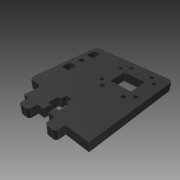
# Autodesk Inventor part: x_motor_cable_mount
Saved by Autodesk Inventor 2014 (Build 180170000, 170)
## iProperties
Created: 2013-12-02
Part Number: x_motor_cable_mount
Material: Plywood, Finish
Document SubType Name: Modeling
Designer: buben
Density: 0.552 g/cm^3
Appearance: Plywood - New
Author: buben
Subject: Laser Cutted
Autodesk Inventor part; units mm, degrees
ref_plane "YZ Plane" through (0, 0, 0) normal (1, 0, 0) x (0, 1, 0)
ref_plane "XZ Plane" through (0, 0, 0) normal (0, 1, 0) x (-1, 0, 0)
ref_plane "XY Plane" through (0, 0, 0) normal (0, 0, 1) x (1, 0, 0)
sketch "Sketch1" plane through (0, 0, 0) normal (0, 0, 1) x (1, 0, 0)
  line L0 (12.2, 0) -> (64.2, 0)
  line L1 (64.2, 0) -> (64.2, 72)
  line L2 (64.2, 72) -> (0, 72)
  line L3 (0, 72) -> (0, 12)
  line L4 (3, 66) -> (9.5, 66)
  line L5 (9.5, 66) -> (9.5, 58)
  line L6 (9.5, 58) -> (3, 58)
  line L7 (3, 58) -> (3, 66)
  line L8 (3, 43) -> (9.5, 43)
  line L9 (9.5, 43) -> (9.5, 35)
  line L10 (9.5, 35) -> (3, 35)
  line L11 (3, 35) -> (3, 43)
  line L12 (0, 12) -> (12.2, 12)
  line L13 (12.2, 12) -> (12.2, 0)
  line L14 (3, 58) -> (9.5, 43) construction
  line L15 (3, 43) -> (9.5, 58) construction
  circle A0 centre (6.25, 50.5) radius 2.25
  point P0 (0, 0)
  dimension "d1" = 6.5
  dimension "d2" = 8
  dimension "d3" = 8
  dimension "d4" = 15
  dimension "d5" = 3
  dimension "d6" = 72
  dimension "d7" = 4.5
  dimension "d8" = 64.2
  dimension "d9" = 12
  dimension "d10" = 52
  dimension "d11" = 6
  constraints: 32 end point, 6 parallel, 5 perpendicular, 3 horizontal, 2 collinear, 1 centre point, 1 horizontal alignment, 1 midpoint, 1 vertical alignment
  measures "d1" distance of L4.start L4.end
  measures "d2" distance of L4.end L5.end
  measures "d3" distance of L8.end L9.end
  measures "d4" distance between parallel lines of L6 L8
  measures "d5" distance between parallel lines of L3 L7
  measures "d6" distance between parallel lines of L0 L2
  measures "d7" diameter of A0
  measures "d8" distance between parallel lines of L1 L3
  measures "d9" distance of L12.end L0.start
  measures "d10" distance of L0.start L0.end
  measures "d11" distance between parallel lines of L2 L4
extrude "Extrusion1" add sketch "Sketch1" along normal blind 6.5
sketch "Sketch2" plane through (0, 0, 6.5) normal (0, 0, 1) x (1, 0, 0)
  line L0 (64.2, 0) -> (64.2, 72) projected
  line L1 (12.2, 0) -> (64.2, 0) projected
  line L2 (29.95, 16.3) -> (34.45, 16.3)
  line L3 (34.45, 0) -> (29.95, 0)
  line L4 (36.95, 12.3) -> (36.95, 5)
  line L5 (27.45, 5) -> (27.45, 12.3)
  line L6 (29.95, 0) -> (29.95, 5)
  line L7 (29.95, 12.3) -> (29.95, 16.3)
  line L8 (27.45, 12.3) -> (29.95, 12.3)
  line L9 (34.45, 12.3) -> (36.95, 12.3)
  line L10 (34.45, 16.3) -> (34.45, 12.3)
  line L11 (34.45, 5) -> (34.45, 0)
  line L12 (36.95, 5) -> (34.45, 5)
  line L13 (29.95, 5) -> (27.45, 5)
  point P0 (0, 0)
  point P1 (32.2, 16.3)
  dimension "d14" = 2.5
  dimension "d15" = 2.5
  dimension "d16" = 4.5
  dimension "d17" = 5
  dimension "d18" = 7.3
  dimension "d19" = 4
  dimension "d20" = 32
  constraints: 24 end point, 10 parallel, 5 collinear, 4 perpendicular, 3 horizontal, 1 midpoint
  measures "d14" distance of L5.end L7.start
  measures "d15" distance of L9.start L4.start
  measures "d16" distance of L2.start L2.end
  measures "d17" distance of L11.start L3.start
  measures "d18" distance of L4.start L4.end
  measures "d19" distance of L2.end L9.start
  measures "d20" distance from line of L0 point (32.2, 16.3)
extrude "Extrusion2" cut sketch "Sketch2" against normal blind 6.5
sketch "Sketch3" plane through (0, 0, 6.5) normal (0, 0, 1) x (1, 0, 0)
  line L0 (34.45, 0) -> (64.2, 0) projected
  line L1 (12.2, 0) -> (29.95, 0) projected
  line L2 (29.95, 16.3) -> (34.45, 16.3) projected
  line L3 (16.7, 0) -> (24.7, 0)
  line L4 (24.7, 0) -> (24.7, -4.5)
  line L5 (22.7, -6.5) -> (18.7, -6.5)
  line L6 (16.7, -4.5) -> (16.7, 0)
  line L7 (39.7, 0) -> (47.7, 0)
  line L8 (47.7, 0) -> (47.7, -4.5)
  line L9 (45.7, -6.5) -> (41.7, -6.5)
  line L10 (39.7, -4.5) -> (39.7, 0)
  arc A0 (16.7, -4.5) -> (18.7, -6.5) centre (18.7, -4.5) ccw
  arc A1 (22.7, -6.5) -> (24.7, -4.5) centre (22.7, -4.5) ccw
  arc A2 (39.7, -4.5) -> (41.7, -6.5) centre (41.7, -4.5) ccw
  arc A3 (45.7, -6.5) -> (47.7, -4.5) centre (45.7, -4.5) ccw
  point P0 (0, 0)
  point P1 (32.2, 16.3)
  dimension "d23" = 2
  dimension "d24" = 8
  dimension "d25" = 8
  dimension "d26" = 6.5
  dimension "d27" = 15
  dimension "d28" = 7.5
  constraints: 16 end point, 8 point on circle, 8 tangent, 4 centre point, 4 parallel, 3 equal radius, 2 horizontal, 2 perpendicular, 2 point on line, 1 collinear, 1 midpoint
  measures "d23" radius of A0
  measures "d24" distance between parallel lines of L4 L6
  measures "d25" distance between parallel lines of L8 L10
  measures "d26" distance between parallel lines of L1 L5
  measures "d27" distance between parallel lines of L10 L4
  measures "d28" distance from line of point (32.2, 16.3) L4
extrude "Extrusion3" add sketch "Sketch3" against normal blind 6.5
chamfer "Chamfer1" distance 2 angle 45 2 edges at (0, 72, 3.25) (64.2, 72, 3.25)
sketch "Sketch4" plane through (0, 0, 0) normal (0, 0, -1) x (-1, 0, 0)
  line L0 (-64.2, 70) -> (-64.2, 0) projected
  line L1 (-2, 72) -> (-62.2, 72) projected
  line L2 (-37.2, 59) -> (-53.2, 59)
  line L3 (-53.2, 59) -> (-53.2, 45)
  line L4 (-53.2, 45) -> (-37.2, 45)
  line L5 (-37.2, 45) -> (-37.2, 59)
  line L6 (-32.2, 66) -> (-58.2, 66) construction
  line L7 (-58.2, 66) -> (-58.2, 38) construction
  line L8 (-58.2, 38) -> (-32.2, 38) construction
  line L9 (-32.2, 38) -> (-32.2, 66) construction
  circle A0 centre (-58.2, 61) radius 1.6
  circle A1 centre (-58.2, 43) radius 1.6
  circle A2 centre (-53.2, 38) radius 1.6
  circle A3 centre (-37.2, 38) radius 1.6
  circle A4 centre (-32.2, 43) radius 1.6
  circle A5 centre (-32.2, 61) radius 1.6
  circle A6 centre (-37.2, 66) radius 1.6
  circle A7 centre (-53.2, 66) radius 1.6
  point P0 (0, 0)
  point P1 (-58.2, 52)
  point P2 (-53.2, 52)
  point P3 (-45.2, 38)
  point P4 (-45.2, 45)
  dimension "d34" = 3.2
  dimension "d35" = 5
  dimension "d36" = 5
  dimension "d37" = 5
  dimension "d38" = 5
  dimension "d39" = 5
  dimension "d40" = 5
  dimension "d41" = 5
  dimension "d42" = 5
  dimension "d43" = 16
  dimension "d44" = 14
  dimension "d45" = 5
  dimension "d46" = 7
  dimension "d47" = 6
  dimension "d48" = 6
  constraints: 16 end point, 8 centre point, 8 point on line, 7 equal radius, 4 midpoint, 4 parallel, 2 horizontal, 2 perpendicular, 1 horizontal alignment, 1 vertical alignment
  measures "d34" diameter of A0
  measures "d35" distance of L6.end A0.centre
  measures "d36" distance of L7.end A1.centre
  measures "d37" distance of A2.centre L7.end
  measures "d38" distance of L8.end A3.centre
  measures "d39" distance of A4.centre L8.end
  measures "d40" distance of L6.start A5.centre
  measures "d41" distance of L6.start A6.centre
  measures "d42" distance of L6.end A7.centre
  measures "d43" distance of L2.start L2.end
  measures "d44" distance of L2.end L3.end
  measures "d45" distance between parallel lines of L9 L5
  measures "d46" distance between parallel lines of L6 L2
  measures "d47" distance between parallel lines of L1 L6
  measures "d48" distance between parallel lines of L0 L7
extrude "Extrusion4" cut sketch "Sketch4" against normal through all
chamfer "Chamfer2" distance 2 angle 45 2 edges at (0, 12, 3.25) (12.2, 12, 3.25)
equation "\"d36\" = d35"
equation "\"d37\" = d35"
equation "\"d38\" = d35"
equation "\"d39\" = d35"
equation "\"d40\" = d35"
equation "\"d41\" = d35"
equation "\"d42\" = d35"
body "Solid1"
